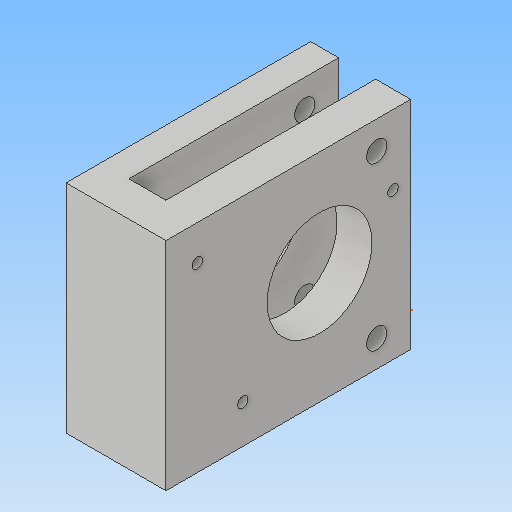
# Autodesk Inventor part: cellSTORM_inverted_spacerblock_KES400
Saved by Autodesk Inventor 2019.4 (Build 234330000, 330)
## iProperties
Created: 2020-12-23
Part Number: cellSTORM_inverted_spacerblock_KES400
Material: Generic
Document SubType Name: Modeling
Designer: diederichbenedict
Density: 1 g/cm^3
Appearance: Default
Author: diederichbenedict
Autodesk Inventor part; units mm, degrees
ref_plane "YZ Plane" through (0, 0, 0) normal (1, 0, 0) x (0, 1, 0)
ref_plane "XZ Plane" through (0, 0, 0) normal (0, 1, 0) x (-1, 0, 0)
ref_plane "Work Plane1" through (0, 0, -31.5) normal (0, -1, 0) x (1, 0, 0)
sketch "Sketch1" plane through (0, 0, -31.5) normal (0, -1, 0) x (1, 0, 0)
  line L0 (0, 31.5) -> (0, 0) projected
  line L1 (5, 26.9723) -> (5, 36.5) projected
  line L2 (-5, 0) -> (-5, 31.5) projected
  line L3 (0, 31.5) -> (-5, 31.5) projected
  line L4 (5, 3.4786) -> (0, 3.4786)
  line L5 (0, 3.4786) -> (0, 38.4786)
  line L6 (0, 38.4786) -> (5, 38.4786)
  line L7 (5, 38.4786) -> (5, 3.4786)
  line L8 (0, 38.4786) -> (-9.3, 38.4786)
  line L9 (-9.3, 38.4786) -> (-9.3, 33.4786)
  line L10 (-9.3, 33.4786) -> (0, 33.4786)
  line L11 (0, 33.4786) -> (0, 38.4786)
  line L12 (-5.3, 3.4786) -> (-9.3, 3.4786)
  line L13 (-9.3, 3.4786) -> (-9.3, 33.4786)
  line L14 (-9.3, 33.4786) -> (-5.3, 33.4786)
  line L15 (-5.3, 33.4786) -> (-5.3, 3.4786)
  dimension "d0" = 35
  dimension "d1" = 5
  dimension "d2" = 4
  dimension "d3" = 0
  dimension "d4" = 0.3
  dimension "d5" = 0
  constraints: 24 end point, 6 parallel, 3 horizontal, 3 perpendicular, 2 point on line
  measures "d0" distance of L4.end L5.end
  measures "d1" distance of L9.end L8.end
  measures "d2" distance of L13.end L14.end
  measures "d3" distance between parallel lines of L13 L9
  measures "d4" distance between parallel lines of L15 L2
  measures "d5" distance between parallel lines of L12 L4
ref_plane "Work Plane2" through (-5, 31, -22.5) normal (0, 1, 0) x (0, 0, 1)
extrude "Extrusion1" add sketch "Sketch1" against normal up to surface (31 mm away)
sketch "Sketch2" plane through (-9.3, 0, -28.0214) normal (-1, 0, 0) x (0, 0, 1)
  arc A0 (11.8709, 3.8471) -> (24.1214, 10.9199) centre (13.0214, 16) ccw projected
  line L0 (11.8709, 3.8471) -> (3.0166, 8.9591) projected
  arc A1 (3.0166, 23.0409) -> (3.0166, 8.9591) centre (13.0214, 16) ccw projected
  line L1 (3.0166, 23.0409) -> (11.5786, 27.9842) projected
  arc A2 (24.1214, 20.7426) -> (11.5786, 27.9842) centre (13.0214, 16) ccw projected
  line L2 (24.1214, 20.7426) -> (24.1214, 10.9199) projected
  line L3 (-3.4786, 32) -> (-3.4786, -6) projected
  line L4 (-3.4786, -6) -> (28.0214, -6) projected
  line L5 (28.0214, -6) -> (28.0214, 32) projected
  line L6 (-3.4786, 32) -> (28.0214, 32) projected
  circle A3 centre (13.0214, 16) radius 7.5
  point P0 (28.0214, 0)
  dimension "d8" = 15
  constraints: 1 centre point, 1 coincident
  measures "d8" diameter of A3
extrude "Extrusion2" cut sketch "Sketch2" against normal through all contours A3
sketch "Sketch3" plane through (5, 0, 6.9786) normal (1, 0, 0) x (0, 0, -1)
  arc A0 (6.1231, 27.7) -> (5.1231, 28.7) centre (5.1231, 27.7) ccw projected
  line L0 (5.1231, 28.7) -> (1.9786, 28.7) projected
  line L1 (1.9786, 28.7) -> (1.9786, 3) projected
  line L2 (1.9786, 3) -> (11.5063, 3) projected
  arc A1 (11.5063, 3) -> (12.5063, 4) centre (11.5063, 4) ccw projected
  line L3 (12.5063, 4) -> (12.5063, 5.8624) projected
  arc A2 (13.5063, 6.8624) -> (12.5063, 5.8624) centre (13.5063, 5.8624) ccw projected
  line L4 (13.5063, 6.8624) -> (31.9786, 6.8624) projected
  line L5 (31.9786, 6.8624) -> (31.9786, 18.397) projected
  arc A3 (32.9786, 19.397) -> (31.9786, 18.397) centre (32.9786, 18.397) ccw projected
  line L6 (32.9786, 19.397) -> (33.9786, 19.397) projected
  arc A4 (33.9786, 19.397) -> (34.9786, 20.397) centre (33.9786, 20.397) ccw projected
  line L7 (34.9786, 20.397) -> (34.9786, 22.9624) projected
  arc A5 (34.9786, 22.9624) -> (33.9786, 23.9624) centre (33.9786, 22.9624) ccw projected
  line L8 (33.9786, 23.9624) -> (7.1231, 23.9624) projected
  arc A6 (6.1231, 24.9624) -> (7.1231, 23.9624) centre (7.1231, 24.9624) ccw projected
  line L9 (6.1231, 24.9624) -> (6.1231, 27.7) projected
  line L10 (14.4786, 22) -> (29.9786, 22) projected
  line L11 (29.9786, 22) -> (29.9786, 8.5) projected
  line L12 (29.9786, 8.5) -> (14.4786, 8.5) projected
  line L13 (14.4786, 8.5) -> (14.4786, 22) projected
  circle A7 centre (4.4786, 26) radius 1 projected
  circle A8 centre (10.9786, 5.5) radius 1 projected
  circle A9 centre (32.4786, 21) radius 1 projected
  point P0 (6.9786, 0)
hole "Hole1" at (5, 5.5, -4) at (5, 26, 2.5) at (5, 21, -25.5) direction (-1, 0, 0) diameter 1.5 end through all
sketch "Sketch4" plane through (-9.3, 0, -28.0214) normal (-1, 0, 0) x (0, 0, 1)
  circle A0 centre (30.5214, 26) radius 0.75 projected
  circle A1 centre (24.0214, 5.5) radius 0.75 projected
  circle A2 centre (2.5214, 21) radius 0.75 projected
  circle A3 centre (13.0214, 16) radius 7.5 projected
  line L0 (35, 31) -> (0, 31) projected
  line L1 (0, 0) -> (0, 31) projected
  line L2 (35, 0) -> (0, 0) projected
  line L3 (35, 0) -> (35, 31) projected
  circle A4 centre (4.8624, 3.8221) radius 1.45
  circle A5 centre (4.8624, 27.0062) radius 1.45
  point P0 (28.0214, 0)
  dimension "d18" = 2.9
  dimension "d19" = 2.9
  constraints: 2 centre point
  measures "d18" diameter of A4
  measures "d19" diameter of A5
extrude "Extrusion3" cut sketch "Sketch4" against normal through all contours A4 | A5
body "Solid1"
